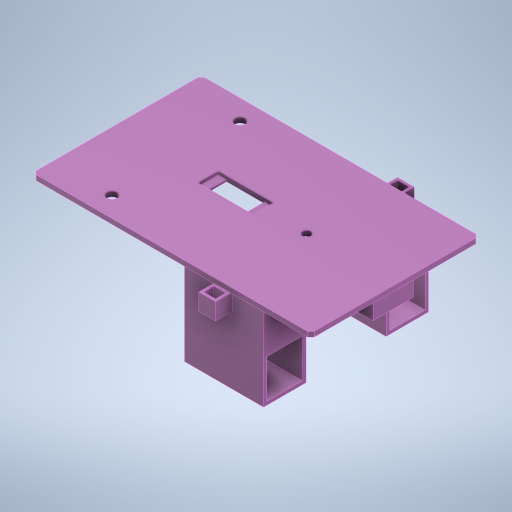
# Autodesk Inventor part: DesainV1.3
Saved by Autodesk Inventor 2024 (Build 280153000, 153)
## iProperties
Created: 2025-12-13
Part Number: DesainV1.3
Material: Generic
Document SubType Name: Modeling
Designer: risda
Density: 1 g/cm^3
Appearance: Smooth - Purple
Author: risda
Autodesk Inventor part; units mm, degrees
ref_plane "YZ Plane" through (0, 0, 0) normal (1, 0, 0) x (0, 1, 0)
ref_plane "XZ Plane" through (0, 0, 0) normal (0, 1, 0) x (-1, 0, 0)
ref_plane "XY Plane" through (0, 0, 0) normal (0, 0, 1) x (1, 0, 0)
sketch "Sketch1" plane through (0, 0, 0) normal (0, 1, 0) x (-1, 0, 0)
  line L0 (0, 0) -> (-165, 0)
  line L1 (-165, 0) -> (-165, 100)
  line L2 (0, 0) -> (0, 100)
  line L3 (0, 100) -> (-165, 100)
  dimension "d0" = 165
  dimension "d1" = 100
  constraints: 8 end point, 2 vertical, 1 horizontal, 1 perpendicular
  measures "d0" distance of L0.start L0.end
  measures "d1" distance of L0.end L1.end
extrude "Extrusion1" add sketch "Sketch1" along normal blind 3
chamfer "Chamfer1" distance 2 angle 45 4 edges at (165, 1.5, 100) (165, 1.5, 0) (0, 1.5, 100) (0, 1.5, 0)
sketch "Sketch2" plane through (0, 0, 0) normal (0, -1, 0) x (1, 0, 0)
  line L0 (163, 100) -> (165, 98) projected
  line L1 (165, 98) -> (135, 98)
  line L2 (135, 98) -> (135, 74.7)
  line L3 (135, 98) -> (90, 98)
  line L4 (135, 74.7) -> (90, 74.7)
  line L5 (90, 74.7) -> (90, 98)
  line L6 (89, 73.7) -> (136, 73.7)
  line L7 (136, 73.7) -> (136, 99)
  line L8 (136, 99) -> (89, 99)
  line L9 (89, 99) -> (89, 73.7)
  line L10 (165, 98) -> (165, 2) projected
  line L11 (165, 2) -> (135, 2)
  line L12 (135, 2) -> (135, 25.3)
  line L13 (135, 25.3) -> (90, 25.3)
  line L14 (90, 25.3) -> (90, 2)
  line L15 (90, 2) -> (135, 2)
  line L16 (136, 26.3) -> (136, 1)
  line L17 (136, 1) -> (89, 1)
  line L18 (89, 1) -> (89, 26.3)
  line L19 (89, 26.3) -> (136, 26.3)
  point P0 (0, 0)
  dimension "d7" = 30
  dimension "d8" = 23.3
  dimension "d9" = 45
  dimension "d10" = 1
  dimension "d11" = 23.3
  dimension "d12" = 1
  dimension "d24" = 45
  constraints: 36 end point, 9 perpendicular, 4 horizontal, 1 point on line, 1 vertical, 6 other
  measures "d7" distance of L0.end L1.end
  measures "d8" distance of L1.end L2.end
  measures "d9" distance of L1.end L3.end
  measures "d10" distance between parallel lines of L4 L6
  measures "d11" distance of L11.end L12.end
  measures "d12" distance between parallel lines of L12 L16
  measures "d24" distance of L14.end L11.end
extrude "Extrusion2" add sketch "Sketch2" along normal blind 50 contours L2 L4 L5 L3 | L7 L6 L9 L8 | L15 L14 L13 L12 | L16 L17 L18 L19
sketch "Sketch3" plane through (136, 0, 99) normal (1, 0, 0) x (0, 0, -1)
  line L0 (72.7, 0) -> (72.7, -50) projected
  line L1 (72.7, -50) -> (72.7, -23)
  line L2 (72.7, -23) -> (98, -23)
  line L3 (98, 0) -> (98, -50) projected
  line L4 (98, -23) -> (98, -50)
  line L5 (98, -50) -> (72.7, -50)
  line L6 (96, -25) -> (74.7, -25)
  line L7 (74.7, -25) -> (74.7, -48)
  line L8 (74.7, -48) -> (96, -48)
  line L9 (96, -48) -> (96, -25)
  line L10 (25.3, 0) -> (25.3, -50) projected
  line L11 (0, -50) -> (25.3, -50)
  line L12 (25.3, -50) -> (25.3, -23)
  line L13 (25.3, -23) -> (0, -23)
  line L14 (0, -23) -> (0, -50)
  line L15 (2, -25) -> (23.3, -25)
  line L16 (23.3, -25) -> (23.3, -48)
  line L17 (23.3, -48) -> (2, -48)
  line L18 (2, -48) -> (2, -25)
  point P0 (99, 0)
  dimension "d15" = 27
  dimension "d16" = 2
  dimension "d17" = 2
  constraints: 32 end point, 6 perpendicular, 4 parallel, 3 point on line, 1 collinear, 1 horizontal, 6 other
  measures "d15" distance of L0.end L1.end
  measures "d16" distance between parallel lines of L2 L6
  measures "d17" distance between parallel lines of L13 L15
extrude "Extrusion3" cut sketch "Sketch3" against normal blind 45.5 contours L9 L8 L7 L6 | L15 L16 L17 L18
sketch "Sketch4" plane through (89, 0, 1) normal (-1, 0, 0) x (0, 0, 1)
  circle A0 centre (12.65, -37.966) radius 2.5
  circle A1 centre (85.35, -40.466) radius 2.5
  point P0 (-1, 0)
  dimension "d20" = 5
  dimension "d21" = 5
  constraints: 2 centre point
  measures "d20" diameter of A0
  measures "d21" diameter of A1
extrude "Extrusion4" cut sketch "Sketch4" against normal blind 41
sketch "Sketch5" plane through (0, 0, 0) normal (0, -1, 0) x (1, 0, 0)
  line L0 (89, 1) -> (89, 26.3) projected
  line L1 (89, 73.7) -> (89, 99) projected
  line L2 (42.1762, 44) -> (98.4238, 44)
  line L3 (70.3, 44) -> (70.3, 56)
  line L4 (70.3, 56) -> (59, 56)
  line L5 (70.3, 56) -> (81.6, 56)
  line L6 (81.6, 56) -> (81.6, 44)
  line L7 (59, 56) -> (59, 44)
  line L8 (59, 50) -> (35, 50)
  line L9 (35, 50) -> (35, 12)
  line L10 (35, 50) -> (35, 88)
  circle A0 centre (35, 12) radius 3.1
  circle A1 centre (35, 88) radius 3.1
  line L11 (89, 73.7) -> (136, 73.7) projected
  line L12 (89, 73.7) -> (71, 73.7)
  point P0 (0, 0)
  point P1 (65, 50)
  point P2 (71, 50)
  point P3 (53.7, 50)
  dimension "d25" = 12
  dimension "d26" = 11.3
  dimension "d27" = 11.3
  dimension "d28" = 24
  dimension "d29" = 38
  dimension "d30" = 38
  dimension "d31" = 6.2
  dimension "d32" = 6.2
  dimension "d39" = 18
  constraints: 20 end point, 3 coincident, 3 point on line, 2 centre point, 2 horizontal, 2 perpendicular, 1 midpoint, 1 vertical
  measures "d25" distance of L3.start L3.end
  measures "d26" distance of L3.end L4.end
  measures "d27" distance of L3.end L5.end
  measures "d28" distance of L8.start L8.end
  measures "d29" distance of L8.end L9.end
  measures "d30" distance of L8.end L10.end
  measures "d31" diameter of A0
  measures "d32" diameter of A1
  measures "d39" distance of L1.start L12.end
extrude "Extrusion5" cut sketch "Sketch5" against normal blind 45.5
sketch "Sketch6" plane through (0, 3, 0) normal (0, 1, 0) x (1, 0, 0)
  line L0 (59, -44) -> (81.6, -44) projected
  line L1 (70.3, -44) -> (70.3, -27.55)
  line L2 (70.3, -44) -> (86.75, -44)
  line L3 (86.75, -44) -> (86.75, -56)
  line L4 (86.75, -56) -> (70.3, -56)
  line L5 (70.3, -56) -> (70.3, -27.55)
  point P0 (0, 0)
  point P1 (71, -38.7)
  dimension "d35" = 16.45
  dimension "d36" = 16.45
  constraints: 10 end point, 3 perpendicular, 1 midpoint, 1 point on line, 1 vertical
  measures "d35" distance of L1.start L1.end
  measures "d36" distance of L1.start L2.end
extrude "Extrusion6" cut sketch "Sketch6" against normal blind 2.1
sketch "Sketch7" plane through (0, 3, 0) normal (0, 1, 0) x (1, 0, 0)
  line L0 (81.6, -44) -> (59, -44) projected
  line L1 (70.3, -44) -> (54.05, -44)
  line L2 (70.3, -44) -> (86.55, -44)
  line L3 (54.05, -44) -> (54.05, -56)
  line L4 (86.75, -56) -> (81.6, -56) projected
  line L5 (54.05, -56) -> (86.75, -56)
  line L6 (86.75, -56) -> (86.55, -44)
  point P0 (0, 0)
  dimension "d40" = 16.25
  dimension "d41" = 16.25
  constraints: 10 end point, 1 horizontal, 1 midpoint, 1 perpendicular, 1 point on line, 1 vertical
  measures "d40" distance of L1.start L1.end
  measures "d41" distance of L1.start L2.end
extrude "Extrusion7" cut sketch "Sketch7" against normal blind 2
sketch "Sketch8" plane through (0, 0, 0) normal (0, -1, 0) x (1, 0, 0)
  line L0 (0, 2) -> (0, 98) projected
  line L1 (0, 50) -> (3, 50)
  line L2 (3, 50) -> (3, 60)
  line L3 (2, 100) -> (163, 100) projected
  line L4 (3, 50) -> (3, 40)
  line L5 (3, 40) -> (8, 40)
  line L6 (8, 40) -> (8, 60)
  line L7 (8, 60) -> (3, 60)
  line L8 (10, 62) -> (10, 38)
  line L9 (10, 38) -> (1, 38)
  line L10 (1, 38) -> (1, 50)
  line L11 (1, 50) -> (1, 62)
  line L12 (1, 62) -> (10, 62)
  point P0 (0, 0)
  dimension "d44" = 3
  dimension "d45" = 10
  dimension "d46" = 10
  dimension "d47" = 5
  dimension "d48" = 2
  constraints: 22 end point, 5 perpendicular, 2 vertical, 1 horizontal, 1 midpoint, 4 other
  measures "d44" distance of L1.start L1.end
  measures "d45" distance of L1.end L2.end
  measures "d46" distance of L1.end L4.end
  measures "d47" distance of L4.end L5.end
  measures "d48" distance between parallel lines of L6 L8
extrude "Extrusion8" add sketch "Sketch8" along normal blind 10
sketch "Sketch9" plane through (89, 0, 99) normal (0, 0, 1) x (1, 0, 0)
  line L0 (47, 0) -> (0, 0) projected
  line L1 (23.5, 0) -> (28.5, 0)
  line L2 (23.5, 0) -> (18.5, 0)
  line L3 (18.5, 0) -> (18.5, -10)
  line L4 (18.5, -10) -> (28.5, -10)
  line L5 (28.5, -10) -> (28.5, 0)
  point P0 (-89, 0)
  dimension "d51" = 5
  dimension "d52" = 5
  dimension "d53" = 10
  constraints: 10 end point, 3 perpendicular, 2 point on line, 1 midpoint
  measures "d51" distance of L1.start L1.end
  measures "d52" distance of L1.start L2.end
  measures "d53" distance of L2.end L3.end
extrude "Extrusion9" add sketch "Sketch9" along normal blind 10
sketch "Sketch10" plane through (107.5, 0, 100) normal (0, 1, 0) x (1, 0, 0)
  line L0 (0, 0) -> (0, -9) projected
  line L1 (10, 0) -> (10, -9) projected
  line L2 (0, 0) -> (10, 0)
  line L3 (10, 0) -> (10, -9)
  line L4 (10, -9) -> (0, -9)
  line L5 (0, -9) -> (0, 0)
  line L6 (1.5, -7.5) -> (8.5, -7.5)
  line L7 (8.5, -7.5) -> (8.5, -1.5)
  line L8 (8.5, -1.5) -> (1.5, -1.5)
  line L9 (1.5, -1.5) -> (1.5, -7.5)
  point P0 (-107.5, 100)
  dimension "d56" = 1.5
  constraints: 16 end point, 7 perpendicular, 3 other
  measures "d56" distance between parallel lines of L4 L6
extrude "Extrusion10" cut sketch "Sketch10" against normal blind 8.5 contours L9 L8 L7 L6
sketch "Sketch11" plane through (136, 0, 1) normal (0, 0, -1) x (-1, 0, 0)
  line L0 (28.5, 0) -> (28.5, -10) projected
  line L1 (28.5, 0) -> (28.5, -10)
  line L2 (18.5, -10) -> (18.5, 0) projected
  line L3 (28.5, -10) -> (18.5, -10)
  line L4 (18.5, -10) -> (18.5, 0)
  line L5 (28.5, 0) -> (18.5, 0)
  point P0 (136, 0)
  constraints: 8 end point, 2 perpendicular, 1 collinear, 1 vertical
extrude "Extrusion11" add sketch "Sketch11" along normal blind 10
sketch "Sketch12" plane through (107.5, 0, 0) normal (0, 1, 0) x (1, 0, 0)
  line L0 (10, 0) -> (0, 0) projected
  line L1 (0, 0) -> (0, 9) projected
  line L2 (0, 0) -> (0, 9)
  line L3 (10, 0) -> (10, 9) projected
  line L4 (0, 9) -> (10, 9)
  line L5 (10, 9) -> (10, 0)
  line L6 (10, 0) -> (0, 0)
  line L7 (8.5, 7.5) -> (1.5, 7.5)
  line L8 (1.5, 7.5) -> (1.5, 1.5)
  line L9 (1.5, 1.5) -> (8.5, 1.5)
  line L10 (8.5, 1.5) -> (8.5, 7.5)
  point P0 (-107.5, 0)
  dimension "d61" = 1.5
  constraints: 16 end point, 5 perpendicular, 1 collinear, 3 other
  measures "d61" distance between parallel lines of L4 L7
extrude "Extrusion12" cut sketch "Sketch12" against normal blind 8.5 contours L10 L9 L8 L7
sketch "Sketch13" plane through (0, 3, 0) normal (0, 1, 0) x (1, 0, 0)
  circle A0 centre (112.58, -50) radius 2.5
  point P0 (0, 0)
  dimension "d64" = 5
  constraints: 1 centre point
  measures "d64" diameter of A0
extrude "Extrusion13" cut sketch "Sketch13" against normal blind 8.5
sketch "Sketch14" plane through (0, 0, 0) normal (0, -1, 0) x (1, 0, 0)
  line L0 (165, 98) -> (165, 2) projected
  line L1 (165, 50) -> (162, 50)
  line L2 (162, 50) -> (162, 40)
  line L3 (162, 50) -> (162, 60)
  line L4 (162, 40) -> (157, 40)
  line L5 (157, 40) -> (157, 60)
  line L6 (157, 60) -> (162, 60)
  line L7 (155, 38) -> (164, 38)
  line L8 (164, 38) -> (164, 50)
  line L9 (164, 50) -> (164, 62)
  line L10 (164, 62) -> (155, 62)
  line L11 (155, 62) -> (155, 38)
  point P0 (0, 0)
  dimension "d67" = 3
  dimension "d68" = 10
  dimension "d69" = 10
  dimension "d70" = 5
  dimension "d71" = 2
  constraints: 22 end point, 4 perpendicular, 2 horizontal, 2 vertical, 1 midpoint, 4 other
  measures "d67" distance of L1.start L1.end
  measures "d68" distance of L1.end L2.end
  measures "d69" distance of L1.end L3.end
  measures "d70" distance of L2.end L4.end
  measures "d71" distance between parallel lines of L4 L7
extrude "Extrusion14" add sketch "Sketch14" along normal blind 10
body "Solid1"
